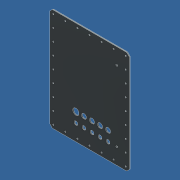
# Autodesk Inventor part: Husky_cover_plate
Saved by Autodesk Inventor 2016 (Build 200138000, 138)
## iProperties
Created: 2021-06-09
Part Number: Husky_cover_plate
Material: Generico
Document SubType Name: Modeling
Designer: Galli Davide
Density: 1 g/cm^3
Appearance: Grigio ferro
Author: Galli Davide
Autodesk Inventor part; units mm, degrees
ref_plane "YZ Plane" through (0, 0, 0) normal (1, 0, 0) x (0, 1, 0)
ref_plane "XZ Plane" through (0, 0, 0) normal (0, 1, 0) x (-1, 0, 0)
ref_plane "XY Plane" through (0, 0, 0) normal (0, 0, 1) x (1, 0, 0)
sketch "Schizzo1" plane through (0, 0, 0) normal (0, 1, 0) x (-1, 0, 0)
  line L0 (0, 0) -> (320, 0)
  line L1 (320, 0) -> (320, -415)
  line L2 (320, -415) -> (0, -415)
  line L3 (0, -415) -> (0, 0)
  dimension "d0" = 320
  dimension "d1" = 415
  constraints: 8 end point, 2 parallel, 1 horizontal, 1 perpendicular
  measures "d0" distance of L1.end L2.end
  measures "d1" distance of L0.end L1.end
extrude "Estrusione1" add sketch "Schizzo1" along normal blind 4
chamfer "Smusso1" distance 10 angle 45 4 edges at (0, 2, 0) (0, 2, -415) (-320, 2, -415) (-320, 2, 0)
sketch "Schizzo2" plane through (0, 4, 0) normal (0, 1, 0) x (1, 0, 0)
  line L0 (-306, 14) -> (-14, 14) construction
  line L1 (-14, 14) -> (-14, 401)
  line L2 (-14, 401) -> (-306, 401) construction
  line L3 (-306, 401) -> (-306, 14) construction
  line L4 (-320, 405) -> (-320, 10) projected
  line L5 (-10, 415) -> (-310, 415) projected
  point P0 (0, 0)
  point P1 (-306, 207.5)
  point P2 (-320, 207.5)
  point P3 (-160, 401)
  point P4 (-160, 415)
  point P5 (-306, 62.375)
  point P6 (-306, 110.75)
  point P7 (-306, 159.125)
  point P8 (-306, 207.5)
  point P9 (-306, 255.875)
  point P10 (-306, 304.25)
  point P11 (-306, 352.625)
  point P12 (-14, 62.375)
  point P13 (-14, 110.75)
  point P14 (-14, 159.125)
  point P15 (-14, 207.5)
  point P16 (-14, 255.875)
  point P17 (-14, 304.25)
  point P18 (-14, 352.625)
  point P19 (-257.3333, 401)
  point P20 (-208.6667, 401)
  point P21 (-160, 401)
  point P22 (-111.3333, 401)
  point P23 (-62.6667, 401)
  point P24 (-257.3333, 14)
  point P25 (-208.6667, 14)
  point P26 (-160, 14)
  point P27 (-111.3333, 14)
  point P28 (-62.6667, 14)
  dimension "d7" = 387
  dimension "d8" = 292
  dimension "d11" = 48.375
  dimension "d18" = 48.375
  dimension "d25" = 48.6667
  dimension "d32" = 48.6667
  constraints: 8 end point, 4 coincident, 4 midpoint, 3 horizontal, 2 parallel, 2 vertical, 1 horizontal alignment, 1 perpendicular, 1 vertical alignment, 24 other
  measures "d7" distance of L2.end L0.start
  measures "d8" distance of L1.end L2.end
  measures "d11" distance of point (-306, 14) point (-306, 62.375)
  measures "d18" distance of point (-14, 14) point (-14, 62.375)
  measures "d25" distance of point (-306, 401) point (-257.333, 401)
  measures "d32" distance of point (-306, 14) point (-257.333, 14)
hole "Foro1" at (-306, 4, -14) at (-14, 4, -14) at (-14, 4, -401) at (-306, 4, -401) at (-306, 4, -62.375) at (-306, 4, -110.75) at (-306, 4, -159.125) at (-306, 4, -207.5) at (-306, 4, -255.875) at (-306, 4, -304.25) at (-306, 4, -352.625) at (-14, 4, -62.375) at (-14, 4, -110.75) at (-14, 4, -159.125) at (-14, 4, -207.5) at (-14, 4, -255.875) at (-14, 4, -304.25) at (-14, 4, -352.625) at (-257.3333, 4, -401) at (-208.6667, 4, -401) at (-160, 4, -401) at (-111.3333, 4, -401) at (-62.6667, 4, -401) at (-257.3333, 4, -14) at (-208.6667, 4, -14) at (-160, 4, -14) at (-111.3333, 4, -14) at (-62.6667, 4, -14) direction (0, -1, 0) diameter 5 end through all
sketch "Schizzo3" plane through (0, 4, 0) normal (0, 1, 0) x (1, 0, 0)
  line L0 (0, 10) -> (0, 405) projected
  line L1 (-310, 0) -> (-10, 0) projected
  line L2 (-10, 415) -> (-310, 415) projected
  point P0 (0, 0)
  point P1 (-50, 65)
  point P2 (-50, 350)
  dimension "d44" = 50
  dimension "d45" = 65
  dimension "d46" = 65
  constraints: 1 vertical alignment
  measures "d44" distance from line of L0 point (-50, 65)
  measures "d45" distance from line of L1 point (-50, 65)
  measures "d46" distance from line of L2 point (-50, 350)
hole "Foro2" at (-50, 4, -65) at (-50, 4, -350) direction (0, -1, 0) diameter 7 end through all
sketch "Schizzo4" plane through (0, 4, 0) normal (0, 1, 0) x (1, 0, 0)
  line L0 (-10, 415) -> (-310, 415) projected
  line L1 (-320, 405) -> (-320, 10) projected
  circle A0 centre (-215, 310) radius 12.5
  arc A1 (-187.5, 318.6603) -> (-177.5, 318.6603) centre (-182.5, 310) ccw
  line L2 (-187.5, 318.6603) -> (-177.5, 318.6603)
  arc A2 (-155, 318.6603) -> (-145, 318.6603) centre (-150, 310) ccw
  line L3 (-155, 318.6603) -> (-145, 318.6603)
  arc A3 (-122.5, 318.6603) -> (-112.5, 318.6603) centre (-117.5, 310) ccw
  line L4 (-122.5, 318.6603) -> (-112.5, 318.6603)
  arc A4 (-90, 318.6603) -> (-80, 318.6603) centre (-85, 310) ccw
  line L5 (-90, 318.6603) -> (-80, 318.6603)
  point P0 (0, 0)
  point P1 (-52.5, 310)
  dimension "d54" = 105
  dimension "d55" = 105
  dimension "d58" = 32.5
  dimension "d63" = 25
  dimension "d64" = 20
  dimension "d65" = 10
  dimension "d70" = 20
  dimension "d71" = 10
  dimension "d76" = 20
  dimension "d77" = 10
  dimension "d88" = 20
  dimension "d89" = 10
  constraints: 8 end point, 8 point on circle, 5 centre point, 5 horizontal, 2 coincident, 5 other
  measures "d54" distance from line of L0 point (-215, 310)
  measures "d55" distance from line of L1 point (-215, 310)
  measures "d58" distance of point (-215, 310) point (-182.5, 310)
  measures "d63" diameter of A0
  measures "d64" diameter of A1
  measures "d65" distance of L2.start L2.end
  measures "d70" diameter of A2
  measures "d71" distance of L3.start L3.end
  measures "d76" diameter of A3
  measures "d77" distance of L4.start L4.end
  measures "d88" diameter of A4
  measures "d89" distance of L5.start L5.end
extrude "Estrusione3" cut sketch "Schizzo4" against normal blind 4
sketch "Schizzo5" plane through (0, 4, 0) normal (0, 1, 0) x (1, 0, 0)
  circle A0 centre (-215, 310) radius 12.5 projected
  line L0 (-10, 415) -> (-310, 415) projected
  arc A1 (-217.5, 357.0711) -> (-212.5, 357.0711) centre (-215, 350) ccw
  line L1 (-217.5, 357.0711) -> (-212.5, 357.0711)
  arc A2 (-185, 357.0711) -> (-180, 357.0711) centre (-182.5, 350) ccw
  line L2 (-185, 357.0711) -> (-180, 357.0711)
  arc A3 (-87.5, 357.0711) -> (-82.5, 357.0711) centre (-85, 350) ccw
  line L3 (-87.5, 357.0711) -> (-82.5, 357.0711)
  arc A4 (-120, 357.0711) -> (-115, 357.0711) centre (-117.5, 350) ccw
  line L4 (-120, 357.0711) -> (-115, 357.0711)
  arc A5 (-152.5, 357.0711) -> (-147.5, 357.0711) centre (-150, 350) ccw
  line L5 (-152.5, 357.0711) -> (-147.5, 357.0711)
  point P0 (0, 0)
  dimension "d94" = 65
  dimension "d97" = 32.5
  dimension "d102" = 15
  dimension "d103" = 5
  dimension "d108" = 15
  dimension "d109" = 5
  dimension "d114" = 15
  dimension "d115" = 5
  dimension "d120" = 15
  dimension "d121" = 5
  dimension "d126" = 15
  dimension "d127" = 5
  constraints: 10 end point, 10 point on circle, 6 horizontal, 5 centre point, 1 coincident, 1 vertical alignment, 4 other
  measures "d94" distance from line of L0 point (-215, 350)
  measures "d97" distance of point (-215, 350) point (-182.5, 350)
  measures "d102" diameter of A1
  measures "d103" distance of L1.start L1.end
  measures "d108" diameter of A2
  measures "d109" distance of L2.start L2.end
  measures "d114" diameter of A3
  measures "d115" distance of L3.start L3.end
  measures "d120" diameter of A4
  measures "d121" distance of L4.start L4.end
  measures "d126" diameter of A5
  measures "d127" distance of L5.start L5.end
extrude "Estrusione4" cut sketch "Schizzo5" against normal blind 4 contours L1 A1 | L2 A2 | L3 A3 | L4 A4 | L5 A5
equation "\"d11\" = 0.125 * d7"
equation "\"d18\" = 0.125 * d7"
equation "\"d25\" = 0.166667 * d8"
equation "\"d32\" = 0.166667 * d8"
